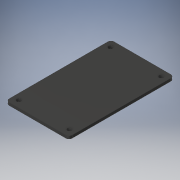
# Autodesk Inventor part: Drok Step Down PCB
Saved by Autodesk Inventor 2019 (Build 230136000, 136)
## iProperties
Created: 2020-02-18
Part Number: Drok Step Down PCB
Material: Generic
Document SubType Name: Modeling
Designer: close
Density: 1 g/cm^3
Appearance: Smooth - Black
Author: close
Autodesk Inventor part; units mm, degrees
ref_plane "YZ Plane" through (0, 0, 0) normal (1, 0, 0) x (0, 1, 0)
ref_plane "XZ Plane" through (0, 0, 0) normal (0, 1, 0) x (-1, 0, 0)
ref_plane "XY Plane" through (0, 0, 0) normal (0, 0, 1) x (1, 0, 0)
sketch "Sketch1" plane through (0, 0, 0) normal (0, 1, 0) x (-1, 0, 0)
  line L0 (1.75, 0) -> (34.25, 0)
  line L1 (36, -1.75) -> (36, -58.25)
  line L2 (34.25, -60) -> (1.75, -60)
  line L3 (0, -58.25) -> (0, -1.75)
  arc A0 (36, -1.75) -> (34.25, 0) centre (34.25, -1.75) ccw
  arc A1 (1.75, 0) -> (0, -1.75) centre (1.75, -1.75) ccw
  arc A2 (0, -58.25) -> (1.75, -60) centre (1.75, -58.25) ccw
  arc A3 (34.25, -60) -> (36, -58.25) centre (34.25, -58.25) ccw
  point P0 (0, 0)
  point P1 (36, -60)
  point P2 (36, 0)
  point P3 (0, -60)
  dimension "d0" = 36
  dimension "d1" = 60
  dimension "d2" = 1.75
  constraints: 8 end point, 8 point on circle, 8 point on line, 8 tangent, 4 centre point, 3 equal radius, 2 parallel, 1 horizontal, 1 perpendicular
  measures "d0" distance of point (36, -60) point (0, -60)
  measures "d1" distance of point (36, 0) point (36, -60)
  measures "d2" radius of A0
extrude "Extrusion1" add sketch "Sketch1" along normal blind 1.6
sketch "Sketch2" plane through (0, 1.6, 0) normal (0, 1, 0) x (1, 0, 0)
  line L0 (-32.5, 3.75) -> (-3.5, 3.75) construction
  line L1 (-3.5, 3.75) -> (-3.5, 56.25) construction
  line L2 (-3.5, 56.25) -> (-32.5, 56.25) construction
  line L3 (-32.5, 56.25) -> (-32.5, 3.75) construction
  line L4 (-36, 58.25) -> (-36, 1.75) projected
  line L5 (0, 1.75) -> (0, 58.25) projected
  line L6 (-1.75, 60) -> (-34.25, 60) projected
  line L7 (-34.25, 0) -> (-1.75, 0) projected
  point P0 (0, 0)
  dimension "d5" = 52.5
  dimension "d6" = 29
  dimension "d7" = 36
  dimension "d8" = 60
  dimension "d9" = 3.75
  dimension "d10" = 3.5
  constraints: 8 end point, 4 coincident, 2 parallel, 1 horizontal, 1 perpendicular
  measures "d5" distance of L2.end L0.start
  measures "d6" distance of L0.start L0.end
  measures "d7" distance between parallel lines of L4 L5
  measures "d8" distance between parallel lines of L6 L7
  measures "d9" distance between parallel lines of L7 L0
  measures "d10" distance between parallel lines of L4 L3
hole "Hole1" at (-32.5, 1.6, -3.75) at (-3.5, 1.6, -3.75) at (-3.5, 1.6, -56.25) at (-32.5, 1.6, -56.25) direction (0, -1, 0) diameter 2.459 depth 8.8 thread size "M3x0.5" class "6H" standard "ANSI Metric M Profile"
equation "\"d9\" = -0.5 * d5 + 0.5 * d8"
equation "\"d10\" = -0.5 * d6 + 0.5 * d7"
body "Solid1"
